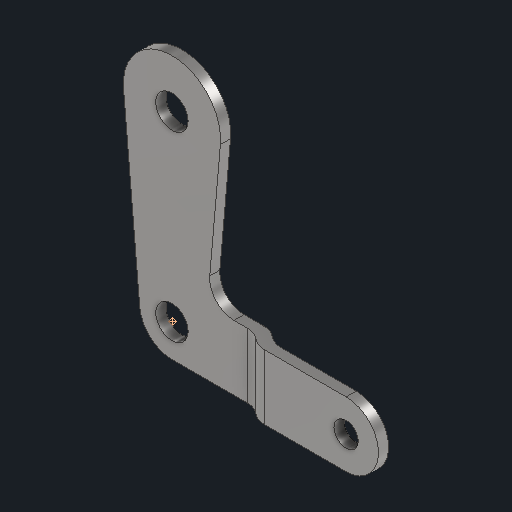
# Autodesk Inventor part: Elbow
Saved by Autodesk Inventor 2025.4 (Build 294407000, 407)
## iProperties
Created: 2026-05-26
Part Number: Elbow
Material: Steel, Mild
Document SubType Name: Modeling
Designer: VuQuan
Density: 7.85 g/cm^3
Appearance: Semi-Polished
Author: VuQuan
Autodesk Inventor part; units mm, degrees
ref_plane "YZ Plane" through (0, 0, 0) normal (1, 0, 0) x (0, 1, 0)
ref_plane "XZ Plane" through (0, 0, 0) normal (0, 1, 0) x (-1, 0, 0)
ref_plane "XY Plane" through (0, 0, 0) normal (0, 0, 1) x (1, 0, 0)
sketch "Sketch1" plane through (0, 0, 0) normal (0, 0, 1) x (1, 0, 0)
  circle A0 centre (0, 0) radius 4
  circle A1 centre (0, 45) radius 4
  circle A2 centre (45.5, 0) radius 3
  line L0 (-7.9683, -0.7111) -> (-11.9525, 43.9333)
  arc A3 (11.9525, 43.9333) -> (-11.9525, 43.9333) centre (0, 45) ccw
  line L1 (11.9525, 43.9333) -> (9.3288, 14.5333)
  arc A4 (9.3288, 14.5333) -> (15.305, 8) centre (15.305, 14) ccw
  line L2 (15.305, 8) -> (45.5, 8)
  line L3 (45.5, -8) -> (0, -8)
  arc A5 (-7.9683, -0.7111) -> (0, -8) centre (0, 0) ccw
  arc A6 (45.5, -8) -> (45.5, 8) centre (45.5, 0) ccw
  dimension "d0" = 8
  dimension "d1" = 6
  dimension "d2" = 45
  dimension "d3" = 45.5
  dimension "d4" = 12
  dimension "d5" = 8
  dimension "d6" = 8
  dimension "d7" = 6
  constraints: 8 end point, 8 point on circle, 8 tangent, 7 centre point, 4 coincident, 2 horizontal alignment, 1 equal radius, 1 parallel, 1 vertical alignment
  measures "d0" diameter of A0
  measures "d1" diameter of A2
  measures "d2" distance of A1.centre point (0, 0)
  measures "d3" distance of A2.centre point (0, 0)
  measures "d4" radius of A3
  measures "d5" radius of A5
  measures "d6" radius of A6
  measures "d7" radius of A4
extrude "Extrusion1" add sketch "Sketch1" along normal mid plane 5
sketch "Sketch3" plane through (0, -8, 2.5) normal (0, -1, 0) x (1, 0, 0)
  line L0 (45.5, -5) -> (45.5, 0) projected
  line L1 (0, 0) -> (45.5, 0) projected
  line L2 (45.5, -5) -> (0, -5) projected
  line L3 (0, -2.5) -> (18.6731, -2.5)
  arc A0 (18.6731, -2.5) -> (21.9803, -1.25) centre (18.6731, 2.5) ccw
  arc A1 (25.2875, 0) -> (21.9803, -1.25) centre (25.2875, -5) ccw
  line L4 (45.5, -2.5) -> (26.8269, -2.5)
  arc A2 (26.8269, -2.5) -> (23.5197, -3.75) centre (26.8269, -7.5) ccw
  arc A3 (20.2125, -5) -> (23.5197, -3.75) centre (20.2125, 0) ccw
  line L5 (23.5197, -3.75) -> (21.9803, -1.25) construction
  line L6 (45.5, -2.5) -> (53.5, -2.5)
  line L7 (53.5, -2.5) -> (53.5, -5)
  line L8 (45.5, 0) -> (45.5, -5) projected
  line L9 (53.5, -5) -> (45.5, -5)
  line L10 (53.5, -5) -> (53.5, 0) projected
  line L11 (12, 0) -> (-12, 0) projected
  line L12 (-12, -5) -> (12, -5) projected
  line L13 (0, -2.5) -> (-12, -2.5)
  line L14 (-12, -5) -> (-12, 0) projected
  line L15 (-12, -5) -> (-12, 0) projected
  line L16 (-12, -5) -> (-12, 0) projected
  point P0 (23.5197, -0.3229)
  point P1 (22.75, -2.5)
  point P2 (22.75, -5)
  point P3 (11.9525, 0)
  point P4 (-11.9525, 0)
  point P5 (11.9525, -5)
  constraints: 14 end point, 9 point on circle, 6 tangent, 4 centre point, 4 horizontal, 4 midpoint, 3 equal radius, 3 point on line, 2 perpendicular, 2 vertical alignment
extrude "Extrusion2" cut sketch "Sketch3" against normal through all contours L2 A3 A2 L4 L0 | L0 L6 L7 L9 | A1 A0 L3 L13 L14 L11 L1
body "Solid1"
